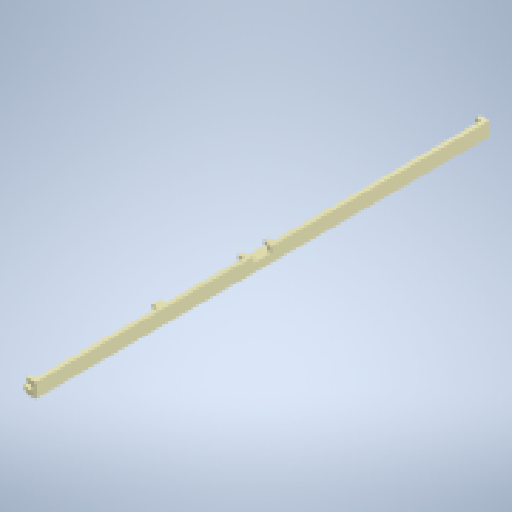
# Autodesk Inventor part: Top Case Rail
Saved by Autodesk Inventor 2025 (Build 290162000, 162)
## iProperties
Created: 2024-07-16
Part Number: Top Case Rail
Material: PET Plastic
Document SubType Name: Modeling
Designer: adam
Density: 1.541 g/cm^3
Appearance: Smooth - Ash
Author: adam
Autodesk Inventor part; units mm, degrees
ref_plane "YZ Plane" through (0, 0, 0) normal (1, 0, 0) x (0, 1, 0)
ref_plane "XZ Plane" through (0, 0, 0) normal (0, 1, 0) x (-1, 0, 0)
ref_plane "XY Plane" through (0, 0, 0) normal (0, 0, 1) x (1, 0, 0)
sketch "Sketch1" plane through (0, 0, 0) normal (0, 0, 1) x (1, 0, 0)
  line L0 (0, 3.75) -> (2, 3.75)
  line L1 (2, 3.75) -> (2, -4)
  line L2 (2, -4) -> (0, -4)
  line L3 (0, -4) -> (0, 3.75) construction
  line L4 (0, -4) -> (-5, -4)
  line L5 (-5, -4) -> (-5, -1)
  line L6 (-5, -1) -> (0, -1)
  line L7 (0, 3.75) -> (-1, 3.75)
  line L8 (-1, 3.75) -> (-1, 0.75)
  line L9 (-1, 0.75) -> (0, 0.75)
  line L10 (0, 0.75) -> (0, 3.75) construction
  line L11 (0, 0.75) -> (0, -1)
  point P0 (0, 0)
  point P1 (0, -0.125)
  point P2 (1, 3.75)
  dimension "d0" = 4
  dimension "d1" = 2
  dimension "d5" = 5
  dimension "d6" = 1.75
  dimension "d7" = 3
  dimension "d11" = 3
  dimension "d12" = 3
  constraints: 24 end point, 5 parallel, 3 horizontal, 3 perpendicular, 2 midpoint, 1 collinear, 1 point on line
  measures "d0" distance from line of L2 point (0, 0)
  measures "d1" distance from line of L1 point (0, -0.125)
  measures "d5" distance between parallel lines of L3 L5
  measures "d6" distance between parallel lines of L6 L9
  measures "d7" distance of L4.end L5.end
  measures "d11" distance between parallel lines of L0 L9
  measures "d12" distance between parallel lines of L1 L8
extrude "Extrusion1" add sketch "Sketch1" along normal blind 245.505
sketch "Sketch2" plane through (-1, 3.75, 245.505) normal (0, 1, 0) x (1, 0, 0)
  line L0 (3, 245.505) -> (3, 0) construction
  line L1 (3, 122.7525) -> (1, 122.7525) construction
  line L2 (1, 245.505) -> (1, 0) construction
  line L3 (3, 127.3525) -> (1, 127.3525)
  line L4 (1, 127.3525) -> (1, 118.1525) construction
  line L5 (1, 118.1525) -> (3, 118.1525) construction
  line L6 (3, 118.1525) -> (3, 127.3525)
  line L7 (3, 122.7525) -> (1, 122.7525) construction
  line L8 (3, 118.1525) -> (1, 118.1525)
  line L9 (1, 127.3525) -> (0, 127.3525)
  line L10 (0, 245.505) -> (0, 0) projected
  line L11 (0, 127.3525) -> (0, 118.1525)
  line L12 (0, 118.1525) -> (1, 118.1525)
  point P0 (0, 118.1525)
  dimension "d13" = 9.2
  constraints: 20 end point, 4 midpoint, 3 perpendicular, 3 point on line, 2 horizontal, 2 parallel, 1 collinear, 1 vertical
  measures "d13" distance of L4.end L3.end
extrude "Extrusion2" cut sketch "Sketch2" against normal up to surface (3 mm away)
sketch "Sketch3" plane through (-1, 0.75, 0) normal (-1, 0, 0) x (0, 0, 1)
  line L0 (118.1525, 0) -> (118.1525, 3) projected
  line L1 (0, 3) -> (118.1525, 3) projected
  line L2 (0, 3) -> (0, 0) projected
  line L3 (0, 0) -> (118.1525, 0) projected
  line L4 (127.3525, 3) -> (127.3525, 0) projected
  line L5 (127.3525, 0) -> (245.505, 0) projected
  line L6 (245.505, 3) -> (245.505, 0) projected
  line L7 (127.3525, 3) -> (245.505, 3) projected
  point P0 (0, -0.75)
extrude "Extrusion3" cut sketch "Sketch3" against normal blind 0.9
chamfer "Chamfer1" distance 2.5 angle 45 1 edges at (-5, -4, 122.7525)
sketch "Sketch4" plane through (-0.1, 0.75, 0) normal (-1, 0, 0) x (0, 0, 1)
  line L0 (0, 3) -> (118.1525, 3) projected
  line L1 (0, 3) -> (2.45, 3)
  line L2 (2.45, 3) -> (2.45, 0.55)
  line L3 (2.45, 0.55) -> (0, 0.55)
  line L4 (0, 0.55) -> (0, 3)
  line L5 (127.3525, 3) -> (245.505, 3) projected
  line L6 (245.505, 3) -> (243.055, 3)
  line L7 (243.055, 3) -> (243.055, 0.55)
  line L8 (243.055, 0.55) -> (245.505, 0.55)
  line L9 (245.505, 0.55) -> (245.505, 3)
  line L10 (0, 3) -> (2.45, 3)
  line L11 (2.45, 3) -> (2.45, 0.55)
  line L12 (245.505, 3) -> (243.055, 3)
  line L13 (243.055, 3) -> (243.055, 0.55)
  point P0 (0, -0.75)
  dimension "d21" = 2.45
  dimension "d22" = 2.45
  dimension "d23" = 2.45
  dimension "d24" = 2.45
  constraints: 24 end point, 7 equal length, 3 perpendicular, 2 horizontal
  measures "d21" distance of L2.end L3.end
  measures "d22" distance of L1.end L2.end
  measures "d23" distance of L7.end L8.end
  measures "d24" distance of L6.end L7.end
extrude "Extrusion4" add sketch "Sketch4" along normal blind 2.95
sketch "Sketch5" plane through (-0.1, 0.75, 0) normal (-1, 0, 0) x (0, 0, 1)
  line L0 (114.505, 2.85) -> (114.505, 0.85) construction
  line L1 (131, 0.85) -> (131, 2.85) construction
  line L2 (131, 2.85) -> (131, 3) construction
  line L3 (127.3525, 3) -> (243.055, 3) construction
  line L4 (114.505, 2.85) -> (114.505, 3) construction
  line L5 (114.505, 3) -> (117.005, 3)
  line L6 (117.005, 3) -> (117.005, 1.05)
  line L7 (117.005, 1.05) -> (114.505, 1.05)
  line L8 (114.505, 1.05) -> (114.505, 3)
  line L9 (131, 3) -> (128.5, 3)
  line L10 (128.5, 3) -> (128.5, 1.05)
  line L11 (128.5, 1.05) -> (131, 1.05)
  line L12 (131, 1.05) -> (131, 3)
  line L13 (2.45, 3) -> (118.1525, 3) projected
  point P0 (0, -0.75)
  dimension "d27" = 2.5
  dimension "d28" = 2.5
  dimension "d29" = 1.95
  constraints: 20 end point, 4 parallel, 2 horizontal, 2 perpendicular, 2 point on line, 2 vertical, 1 collinear
  measures "d27" distance of L6.end L7.end
  measures "d28" distance of L10.end L11.end
  measures "d29" distance of L9.end L10.end
extrude "Extrusion5" add sketch "Sketch5" along normal blind 2.95
sketch "Sketch6" plane through (-0.1, 0.75, 0) normal (-1, 0, 0) x (0, 0, 1)
  line L0 (172.5025, 2.85) -> (172.5025, 0.85) construction
  line L1 (177.6025, 0.85) -> (177.6025, 2.85) construction
  line L2 (177.6025, 2.85) -> (177.6025, 3) construction
  line L3 (131, 3) -> (243.055, 3) construction
  line L4 (172.5025, 2.85) -> (172.5025, 3) construction
  line L5 (172.7025, 3) -> (177.4025, 3)
  line L6 (177.4025, 3) -> (177.4025, 1.05)
  line L7 (177.4025, 1.05) -> (172.7025, 1.05)
  line L8 (172.7025, 1.05) -> (172.7025, 3)
  point P0 (0, -0.75)
  dimension "d32" = 0.2
  dimension "d33" = 0.2
  dimension "d34" = 1.95
  constraints: 12 end point, 3 parallel, 3 point on line, 1 horizontal, 1 perpendicular, 1 vertical
  measures "d32" distance between parallel lines of L8 L0
  measures "d33" distance between parallel lines of L6 L2
  measures "d34" distance between parallel lines of L3 L7
extrude "Extrusion6" add sketch "Sketch6" along normal blind 2.95
body "Solid1"
